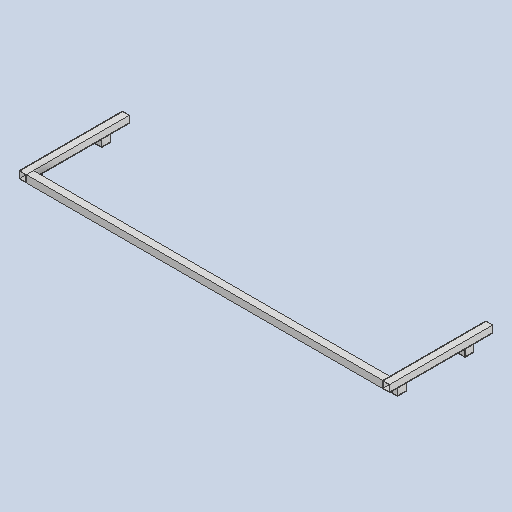
# Autodesk Inventor part: PernasMesa
Saved by Autodesk Inventor 2025 (Build 290162000, 162)
## iProperties
Created: 2022-08-17
Part Number: PernasMesa
Material: Generic
Document SubType Name: Modeling
Designer: cvss2
Density: 1 g/cm^3
Appearance: Default
Author: cvss2
Autodesk Inventor part; units mm, degrees
ref_plane "YZ Plane" through (0, 0, 0) normal (1, 0, 0) x (0, 1, 0)
ref_plane "XZ Plane" through (0, 0, 0) normal (0, 1, 0) x (-1, 0, 0)
ref_plane "XY Plane" through (0, 0, 0) normal (0, 0, 1) x (1, 0, 0)
sketch "Sketch1" plane through (0, 0, 0) normal (0, 1, 0) x (-1, 0, 0)
  line L0 (0, 0) -> (-2608, 0)
  line L1 (-2608, 0) -> (-2608, 725)
  line L2 (-2608, 725) -> (0, 725)
  line L3 (0, 725) -> (0, 0)
  line L4 (-50, 675) -> (-2558, 675)
  line L5 (-2558, 675) -> (-2558, 50)
  line L6 (-2558, 50) -> (-50, 50)
  line L7 (-50, 50) -> (-50, 675)
  line L8 (-2558, 675) -> (-2558, 725)
  line L9 (-2558, 50) -> (-2558, 0)
  line L10 (-50, 50) -> (-50, 0)
  line L11 (-50, 675) -> (-50, 725)
  line L12 (-50, 250) -> (-2558, 250)
  dimension "d0" = 2608
  dimension "d1" = 725
  dimension "d2" = 50
  dimension "d7" = 250
  constraints: 26 end point, 10 point on line, 4 parallel, 3 perpendicular, 1 horizontal, 3 other
  measures "d0" distance of L1.end L2.end
  measures "d1" distance of L0.end L1.end
  measures "d2" distance between parallel lines of L2 L4
  measures "d7" distance between parallel lines of L0 L12
extrude "Extrusion1" add sketch "Sketch1" against normal blind 50 contours L0 L10 L7 L11 L2 L3 | L0 L1 L2 L8 L5 L9
extrude "Extrusion2" add sketch "Sketch1" against normal blind 50 separate body contours L11 L4 L8 L2
shell "Shell1" thickness 3 removed faces 4 at (16.6667, -16.6667, 725) at (33.3333, -16.6667, 0) at (2574.6667, -16.6667, 725) at (2591.3333, -16.6667, 0) bodies 1
sketch "Sketch3" plane through (0, -50, 0) normal (0, -1, 0) x (1, 0, 0)
  line L0 (50, 725) -> (0, 725) projected
  line L1 (0, 725) -> (0, 0) projected
  line L2 (0, 0) -> (50, 0) projected
  line L3 (50, 0) -> (50, 725) projected
  line L4 (2558, 0) -> (2608, 0) projected
  line L5 (2608, 0) -> (2608, 725) projected
  line L6 (2608, 725) -> (2558, 725) projected
  line L7 (2558, 725) -> (2558, 0) projected
  line L8 (0, 0) -> (0, 725) projected
  line L9 (0, 670) -> (50, 670)
  line L10 (50, 670) -> (50, 610)
  line L11 (50, 610) -> (0, 610)
  line L12 (0, 610) -> (0, 670)
  line L13 (2558, 670) -> (2608, 670)
  line L14 (2608, 670) -> (2608, 610)
  line L15 (2608, 610) -> (2558, 610)
  line L16 (2558, 610) -> (2558, 670)
  line L17 (0, 195) -> (50, 195)
  line L18 (50, 195) -> (50, 135)
  line L19 (50, 135) -> (0, 135)
  line L20 (0, 135) -> (0, 195)
  line L21 (2558, 195) -> (2608, 195)
  line L22 (2608, 195) -> (2608, 135)
  line L23 (2608, 135) -> (2558, 135)
  line L24 (2558, 135) -> (2558, 195)
  point P0 (0, 135)
  point P1 (0, 610)
  dimension "d28" = 50
  dimension "d29" = 60
  dimension "d30" = 55
  dimension "d33" = 2558
  dimension "d36" = 475
  constraints: 32 end point, 2 horizontal, 2 parallel, 1 perpendicular, 1 point on line, 1 vertical, 24 other
  measures "d28" distance of L10.end L11.end
  measures "d29" distance of L9.end L10.end
  measures "d30" distance between parallel lines of L0 L9
  measures "d33" distance of L9.start L13.start
  measures "d36" distance of L9.start L17.start
extrude "Extrusion4" add sketch "Sketch3" along normal blind 50 separate body contours L3 L11 L1 L9 | L3 L19 L1 L17 | L7 L21 L5 L23 | L7 L13 L5 L15
shell "Shell3" thickness 3 removed faces 8 at (33.3333, -66.6667, 670) at (33.3333, -66.6667, 195) at (2591.3333, -66.6667, 195) at (2591.3333, -66.6667, 670) at (16.6667, -66.6667, 610) at (16.6667, -66.6667, 135) at (2574.6667, -66.6667, 135) at (2574.6667, -66.6667, 610) bodies 3
body "Solid1"
body "Solid2"
body "Solid4"
